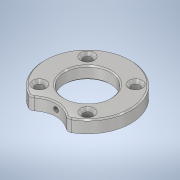
# Autodesk Inventor part: Motor Mount
Saved by Autodesk Inventor 2020.1 (Build 241239000, 239)
## iProperties
Created: 2019-03-01
Part Number: Motor Mount
Material: Aluminum 6061-AHC
Document SubType Name: Modeling
Designer: Petar
Density: 2.7 g/cm^3
Appearance: Aluminum - Dark
Mass: 6.25091 g
Surface Area: 19.0882 cm^2
Volume: 2.31515 cm^3
Author: Petar
Autodesk Inventor part; units mm, degrees
ref_plane "YZ Plane" through (0, 0, 0) normal (1, 0, 0) x (0, 1, 0)
ref_plane "XZ Plane" through (0, 0, 0) normal (0, 1, 0) x (-1, 0, 0)
sketch "Sketch1" plane through (0, 0, 0) normal (0, 1, 0) x (-1, 0, 0)
  circle A0 centre (0, 0) radius 9.25
  circle A1 centre (0, 0) radius 13.75 construction
  circle A2 centre (9.7227, -9.7227) radius 1.65
  line L0 (9.7227, -9.7227) -> (0, 0) construction
  circle A3 centre (9.7227, 9.7227) radius 1.65
  circle A4 centre (-9.7227, 9.7227) radius 1.65
  circle A5 centre (-9.7227, -9.7227) radius 1.65
  line L1 (0, 0) -> (0, -13.75) construction
  circle A6 centre (0, 0) radius 17.5
  circle A7 centre (0, 0) radius 9.5 construction
  line L2 (7.5, 15.8114) -> (0, 9.5) construction
  line L3 (0, 9.5) -> (-7.5, 15.8114) construction
  spline S0 degree 2 poles (7.5, 15.8114) (0, 9.5) (-7.5, 15.8114) knots 1 1 1 2 2 2
  line L4 (7.5, 15.8114) -> (-7.5, 15.8114) construction
  line L5 (0, 9.5) -> (0, 9.5) construction
  dimension "d10" = 19
  dimension "d0" = 18.5
  dimension "d2" = 3.3
  dimension "d6" = 360
  dimension "d8" = 45
  dimension "d11" = 15
  dimension "d27" = 0
  dimension "d30" = 8
  dimension "d36" = 27.5
  constraints: 8 end point, 7 centre point, 5 coincident, 5 point on circle, 2 vertical, 1 collinear, 1 horizontal, 1 vertical alignment, 15 other
  measures "d0" diameter of A0
  measures "d2" diameter of A2
  measures "d8" angle of L1 L0
  measures "d11" distance of L2.start L4.end
  measures "d27" distance of L5.start L5.end
  measures "d36" diameter of A1
extrude "Extrusion1" add sketch "Sketch1" along normal blind 5 contours A6 S0 picked at (12.2171, -4.8968)
fillet "Fillet1" radius 2 2 edges at (-7.5, 2.5, 15.8114) (7.5, 2.5, 15.8114)
fillet "Fillet2" [suppressed]
chamfer "Chamfer1" distance 0.5 angle 45 2 edges at (9.25, 5, 0) (9.25, 0, 0)
chamfer "Chamfer2" distance 0.5 angle 45 4 edges at (0, 5, -17.5) (-7.6088, 5, 15.4375) (0, 5, 12.6557) (7.6088, 5, 15.4375)
chamfer "Chamfer3" distance 1.1 angle 45 4 edges at (-8.0727, 5, 9.7227) (-8.0727, 5, -9.7227) (11.3727, 5, 9.7227) (11.3727, 5, -9.7227)
ref_plane "Work Plane1" through (0, 2.5, 12.6557) normal (0, 0, 1) x (1, 0, 0)
sketch "Sketch2" plane through (0, 2.5, 12.6557) normal (0, 0, 1) x (1, 0, 0)
  line L0 (9.75, 2.5) -> (-9.75, 2.5) construction
  line L1 (-8.4673, 2.5) -> (8.4673, 2.5) construction
  line L2 (-6.833, 2.5) -> (-8.4673, 2.5) construction
  line L3 (6.833, 2.5) -> (-6.833, 2.5) construction
  line L4 (8.4673, 2.5) -> (6.833, 2.5) construction
  line L5 (12.4727, 2.5) -> (6.9727, 2.5) construction
  line L6 (12.4727, 2.5) -> (6.9727, 2.5) construction
  line L7 (-6.9727, 2.5) -> (-12.4727, 2.5) construction
  line L8 (-6.9727, 2.5) -> (-12.4727, 2.5) construction
  line L9 (-8.0727, -2.5) -> (-11.3727, -2.5) construction
  line L10 (-8.0727, -2.5) -> (-11.3727, -2.5) construction
  line L11 (11.3727, -2.5) -> (8.0727, -2.5) construction
  line L12 (11.3727, -2.5) -> (8.0727, -2.5) construction
  line L13 (6.5373, -2.5) -> (8.7163, -2.5) construction
  line L14 (-6.5373, -2.5) -> (6.5373, -2.5) construction
  line L15 (-8.7163, -2.5) -> (-6.5373, -2.5) construction
  line L16 (8.7163, -2.5) -> (-8.7163, -2.5) construction
  line L17 (-9.75, -2.5) -> (9.75, -2.5) construction
  line L18 (0, -2.5) -> (0, 2.5) construction
  line L19 (9.75, 2.5) -> (-9.75, 2.5) construction
  circle A0 centre (0, 0) radius 1.25
  dimension "d40" = 2.5
  dimension "d41" = 5
  dimension "d42" = 2.5
  constraints: 2 end point, 1 centre point, 1 midpoint, 2 other
  measures "d40" diameter of A0
  measures "d41" distance between parallel lines of L14 L3
  measures "d42" distance from line of L14 A0.centre
hole "Hole1" at (0, 2.5, 12.6557) direction (0, 0, 1) diameter 2 depth 8 start extended yes
thread "Thread5" size "M2x0.4" class "6H" standard "ANSI Metric M Profile" full length
equation "\"d42\" = 0.5 * d41"
body "Solid1"
